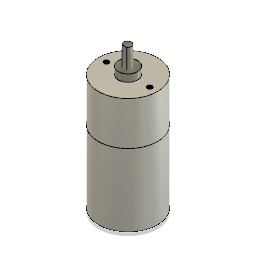
MotorBracket v27 (Autodesk Fusion 360 archive; units mm, degrees)
design "Motor"
Autodesk Fusion 360 part; units mm, degrees
sketch "Sketch1" plane through (0, 0, 0) normal (0, 1, 0) x (1, 0, 0)
  circle A0 centre (0, 0) radius 12.25
  dimension "d1" = 24.5
  measures "d1" diameter of A0
extrude "Extrude1" add sketch "Sketch1" along normal blind 30 makes body 1
sketch "Sketch2" plane through (0, 0, 0) normal (0, 1, 0) x (1, 0, 0)
  circle A0 centre (0, 0) radius 12.25
extrude "Extrude2" add sketch "Sketch2" along normal blind 18 separate body makes body 2
move_body "Move1" bodies 2 to x (1, 0, 0) y (0, 1, 0) z (0, 0, 1) at (0, 30, 0)
sketch "Sketch3" plane through (0, 0, 0) normal (0, 1, 0) x (1, 0, 0)
  circle A0 centre (30, 0) radius 4
  dimension "d6" = 8
  measures "d6" diameter of A0
extrude "Extrude3" add sketch "Sketch3" along normal blind 3 separate body makes body 3
move_body "Move2" bodies 3 to x (1, 0, 0) y (0, 1, 0) z (0, 0, 1) at (-30, 48, 0)
sketch "Sketch5" plane through (0, 0, 0) normal (0, 1, 0) x (1, 0, 0)
  arc A0 (-28, 0) -> (-30, 0) centre (-29, 1.3333) ccw
  line L0 (-30, 0) -> (-28, 0)
extrude "Extrude5" add sketch "Sketch5" along normal blind 14 separate body makes body 4
move_body "Move4" bodies 4 to x (1, 0, 0) y (0, 1, 0) z (0, 0, 1) at (29, 45, 1)
move_body "Move5" bodies 4 to x (1, 0, 0) y (0, 1, 0) z (0, 0, 1) at (0, 0, 0.5)
sketch "Sketch6" plane through (0, 0, 0) normal (0, 1, 0) x (1, 0, 0)
  circle A0 centre (0, 0) radius 11.5
  dimension "d14" = 23
  measures "d14" diameter of A0
extrude "Extrude6" cut sketch "Sketch6" along normal blind 1.2 bodies 1
sketch "Sketch7" plane through (0, 1.2, 0) normal (0, -1, 0) x (1, 0, 0)
  circle A0 centre (0, 0) radius 11.5
  circle A1 centre (0, 0) radius 4
extrude "Extrude7" add sketch "Sketch7" along normal blind 1.7 contours A1 bodies 1
fillet "Fillet1" radius 0.5 1 edges at (-3.7293, -0.5, -1.4465) on bodies 1
fillet "Fillet2" radius 1 1 edges at (-10.7218, 1.2, 4.1586) on bodies 1
sketch "Sketch8" plane through (0, 0, 0) normal (1, 0, 0) x (0, 0, -1)
  arc A0 (-8, -4) -> (-6, -4) centre (-7, -4) ccw
  arc A1 (6, -4) -> (8, -4) centre (7, -4) ccw
  line L0 (-8, -4) -> (-8, -2)
  line L1 (-8, -2) -> (-6, -2)
  line L2 (-6, -2) -> (-6, -4)
  line L3 (6, -4) -> (6, -2)
  line L4 (6, -2) -> (8, -2)
  line L5 (8, -2) -> (8, -4)
  circle A2 centre (-7, -4) radius 0.5
  circle A3 centre (7, -4) radius 0.5
extrude "Extrude8" add sketch "Sketch8" along normal blind 0.5 separate body makes body 5 at (0, -2.5005, 7.0125) makes body 6 at (0, -2.5005, -6.9875)
move_body "Move6" bodies 5 6 to x (1, 0, 0) y (0, 1, 0) z (0, 0, 1) at (0, 3.5, 0)
move_body "Move7" bodies 5 to x (0, 0, -1) y (0, 1, 0) z (1, 0, 0) at (-6, 0, 6)
move_body "Move8" bodies 6 to x (0, 0, -1) y (0, 1, 0) z (1, 0, 0) at (7, 0, -8)
move_body "Move9" bodies 5 to x (1, 0, 0) y (0, 1, 0) z (0, 0, 1) at (-1, 0, 3)
move_body "Move10" bodies 5 to x (1, 0, 0) y (0, 1, 0) z (0, 0, 1) at (0, 0, -0.5)
sketch "Sketch9" plane through (0, 51, 0) normal (0, 1, 0) x (-1, 0, 0)
  circle A0 centre (0, 0) radius 4
  circle A1 through (10, 0, -3) (8.5, 0.866, -3) (8.5, -0.866, -3)
  circle A2 through (-8, 0, -3) (-9.5, 0.866, -3) (-9.5, -0.866, -3)
extrude "Extrude9" cut sketch "Sketch9" against normal blind 4 contours A1 | A2 in plane through (0, 48, 0) normal (0, 1, 0) bodies 2
thread "Thread1" "ISO Metric profile 2.0 M2x0.4 6H" major diameter 2.074 minor diameter 1.623 pitch 0.4 angle 60 modelled right hand crest width 0.05 on face at (-9.995, 46.6667, -0.0996) crest through (-9.8115, 48.225, 0) on face at (8.005, 46.6667, -0.0996) crest through (8.1885, 48.225, 0) on bodies 2
named bodies: "Motor", "Gearbox", "Bush", "Spindle", "PveTerminal", "NveTerminal"
